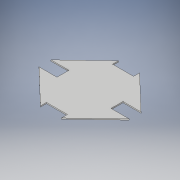
# Autodesk Inventor part: Wood Base
Saved by Autodesk Inventor 2018 (Build 220112000, 112)
## iProperties
Created: 2019-01-03
Part Number: Wood Base
Material: Generic
Document SubType Name: Modeling
Designer: Gabriel
Density: 1 g/cm^3
Appearance: Default
Author: Gabriel
Autodesk Inventor part; units mm, degrees
ref_plane "YZ Plane" through (0, 0, 0) normal (1, 0, 0) x (0, 1, 0)
ref_plane "XZ Plane" through (0, 0, 0) normal (0, 1, 0) x (-1, 0, 0)
ref_plane "XY Plane" through (0, 0, 0) normal (0, 0, 1) x (1, 0, 0)
sketch "Sketch1" plane through (0, 0, 0) normal (0, 1, 0) x (-1, 0, 0)
  line L0 (-212.3768, -1157.61) -> (-364.7768, -1157.61)
  line L1 (-364.7768, -1157.61) -> (-364.7768, -1259.21)
  line L2 (-364.7768, -1259.21) -> (-212.3768, -1259.21)
  line L3 (-974.3768, -1157.61) -> (-821.9768, -1157.61)
  line L4 (-821.9768, -1157.61) -> (-821.9768, -1259.21)
  line L5 (-821.9768, -1259.21) -> (-974.3768, -1259.21)
  line L6 (-682.2768, -929.01) -> (-504.4768, -929.01)
  line L7 (-682.2768, -1487.81) -> (-504.4768, -1487.81)
  line L8 (-504.4768, -1487.81) -> (-504.4768, -1538.61)
  line L9 (-682.2768, -1487.81) -> (-682.2768, -1538.61)
  line L10 (-504.4768, -929.01) -> (-504.4768, -878.21)
  line L11 (-682.2768, -929.01) -> (-682.2768, -878.21)
  line L12 (-212.3768, -1259.21) -> (-504.4768, -1538.61)
  line L13 (-974.3768, -1157.61) -> (-682.2768, -878.21)
  line L14 (-504.4768, -878.21) -> (-212.3768, -1157.61)
  line L15 (-682.2768, -1538.61) -> (-974.3768, -1259.21)
  dimension "d9" = 152.4
  dimension "d10" = 101.6
  dimension "d14" = 152.4
  dimension "d15" = 101.6
  dimension "d27" = 177.8
  dimension "d29" = 177.8
  dimension "d30" = 50.8
  dimension "d31" = 50.8
  dimension "d32" = 50.8
  constraints: 32 end point, 4 perpendicular, 4 vertical, 1 horizontal, 1 parallel, 1 point on line
  measures "d9" distance of L0.start L0.end
  measures "d10" distance of L0.end L1.end
  measures "d14" distance of L3.start L3.end
  measures "d15" distance of L3.end L4.end
  measures "d27" distance of L6.start L6.end
  measures "d29" distance of L7.start L7.end
  measures "d30" distance of L7.end L8.end
  measures "d31" distance of L7.start L9.end
  measures "d32" distance of L6.end L10.end
extrude "Wood Base" add sketch "Sketch1" along normal blind 9.525
body "Solid2"
